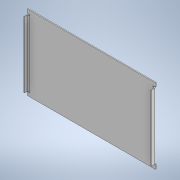
# Autodesk Inventor part: Fondo
Saved by Autodesk Inventor 2021 (Build 250183000, 183)
## iProperties
Created: 2021-07-21
Part Number: Fondo
Material: Generic
Document SubType Name: Sheet Metal
Designer: admin
Density: 1 g/cm^3
Sheet Metal Rule: Por defecto_mm
Appearance: Default
Flat Pattern Width: 41 cm
Flat Pattern Length: 73.2619 cm
Flat Pattern Area: 3003.74 cm^2
Sheet Metal Width: 0.410 m
Sheet Metal Length: 0.733 m
Sheet Metal Area: 0.300 m^2
Author: admin
Autodesk Inventor part; units mm, degrees
note: some values were not read from the file. Chosen so that the rebuilt part matches the saved one: relief shape of "Placa2"; relief shape of "Placa3".
ref_plane "YZ Plane" through (0, 0, 0) normal (1, 0, 0) x (0, 1, 0)
ref_plane "XZ Plane" through (0, 0, 0) normal (0, 1, 0) x (-1, 0, 0)
ref_plane "XY Plane" through (0, 0, 0) normal (0, 0, 1) x (1, 0, 0)
sketch "Boceto1" plane through (0, 0, 0) normal (0, 0, 1) x (1, 0, 0)
  line L0 (-350, 205) -> (350, 205)
  line L1 (350, 205) -> (350, -205)
  line L2 (350, -205) -> (-350, -205)
  line L3 (-350, -205) -> (-350, 205)
  line L4 (-350, 205) -> (350, -205) construction
  line L5 (350, 205) -> (-350, -205) construction
  point P0 (0, 0)
  dimension "d0" = 700
  dimension "d1" = 410
  measures "d0" distance of L1.end L2.end
  measures "d1" distance of L0.end L1.end
extrude "Placa1" add sketch "Boceto1" along normal blind 5
sketch "Boceto2" plane through (-345, -205, 0) normal (-1, 0, 0) x (0, -1, 0)
  line L0 (-385, 0) -> (-25, 0)
  line L1 (-25, 0) -> (-25, 25)
  line L2 (-25, 25) -> (-385, 25)
  line L3 (-385, 25) -> (-385, 0)
  constraints: 8 end point
edge flange "Pestaña1" height 25 angle 90 thickness 5 bend radius 5 thickness toward (-1, 0, 0) relief straight relief width 5 relief depth 2.5 edges at (-350, 0, 5) wall of the first edge with corners at (-345, 180, 0) (-345, -180, 0) (-345, -180, 25) (-345, 180, 25)
bend "Doblez1"
corner "Esquina1"
sketch "Boceto3" plane through (345, 205, 0) normal (1, 0, 0) x (0, 1, 0)
  line L0 (-385, 0) -> (-25, 0)
  line L1 (-25, 0) -> (-25, 25)
  line L2 (-25, 25) -> (-385, 25)
  line L3 (-385, 25) -> (-385, 0)
  constraints: 8 end point
edge flange "Pestaña2" height 25 angle 90 thickness 5 bend radius 5 thickness toward (1, 0, 0) relief straight relief width 5 relief depth 2.5 edges at (350, 0, 5) wall of the first edge with corners at (345, -180, 0) (345, 180, 0) (345, 180, 25) (345, -180, 25)
bend "Doblez2"
corner "Esquina2"
equation "\"d2\" = Thickness"
equation "\"d3\" = BendReliefWidth"
equation "\"d4\" = BendReliefDepth"
equation "\"d5\" = MinimumRemnant"
equation "\"d6\" = TransitionRadius"
equation "\"d10\" = BendRadius"
equation "\"d11\" = CornerReliefSize"
equation "\"d12\" = GapSize"
equation "\"d13\" = JacobiRadiusSize"
equation "\"d14\" = BendReliefWidth"
equation "\"d15\" = BendReliefDepth"
equation "\"d16\" = MinimumRemnant"
equation "\"d17\" = TransitionRadius"
equation "\"d21\" = BendRadius"
equation "\"d22\" = CornerReliefSize"
equation "\"d23\" = GapSize"
equation "\"d24\" = JacobiRadiusSize"
equation "\"BendRadius\" = Thickness"
equation "\"BendReliefWidth\" = Thickness"
equation "\"BendReliefDepth\" = 0.5 * Thickness"
equation "\"TransitionRadius\" = BendRadius"
equation "\"JacobiRadiusSize\" = BendRadius"
equation "\"GapSize\" = Thickness"
equation "\"Thickness\" = 5"
equation "\"MinimumRemnant\" = 10"
equation "\"CornerReliefSize\" = 20"
